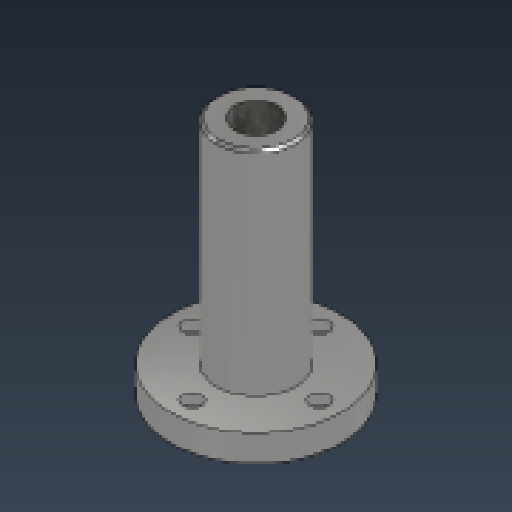
# Autodesk Inventor part: Łożysko liniowe z kołnierzem okrągłym LMF08UU-L
Saved by Autodesk Inventor 2025.2 (Build 292293000, 293)
## iProperties
Created: 2025-04-13
Part Number: Łożysko liniowe z kołnierzem okrągłym LMF08UU-L
Material: Stainless Steel
Document SubType Name: Modeling
Designer: Kacper Mik
Density: 8 g/cm^3
Appearance: Semi-Polished
Mass: 67.1779 g
Surface Area: 52.807 cm^2
Volume: 8.39724 cm^3
Author: Kacper Mik
Autodesk Inventor part; units mm, degrees
ref_plane "YZ Plane" through (0, 0, 0) normal (1, 0, 0) x (0, 1, 0)
ref_plane "XZ Plane" through (0, 0, 0) normal (0, 1, 0) x (-1, 0, 0)
ref_plane "XY Plane" through (0, 0, 0) normal (0, 0, 1) x (1, 0, 0)
sketch "Sketch1" plane through (0, 0, 0) normal (0, 1, 0) x (-1, 0, 0)
  circle A0 centre (0, 0) radius 16
  dimension "d0" = 32
  constraints: 1 centre point, 1 coincident
  measures "d0" diameter of A0
extrude "Extrusion1" add sketch "Sketch1" along normal blind 5
sketch "Sketch2" plane through (0, 5, 0) normal (0, 1, 0) x (1, 0, 0)
  circle A0 centre (0, 0) radius 7.5
  dimension "d3" = 15
  constraints: 1 centre point, 1 coincident
  measures "d3" diameter of A0
extrude "Extrusion2" add sketch "Sketch2" along normal blind 40
sketch "Sketch3" plane through (0, 0, 0) normal (0, -1, 0) x (1, 0, 0)
  circle A0 centre (0, 0) radius 12 construction
  point P0 (0, 12)
  point P1 (12, 0)
  point P2 (0, -12)
  point P3 (-12, 0)
  dimension "d6" = 24
  constraints: 4 point on circle, 2 horizontal alignment, 2 vertical alignment, 1 centre point, 1 coincident
  measures "d6" diameter of A0
hole "Hole1" at (0, 0, 12) at (12, 0, 0) at (0, 0, -12) at (-12, 0, 0) direction (0, 1, 0) diameter 3.5 end through all counterbore diameter 6 counterbore depth 3.1 clearance for "Hex Head Cap Screw ISO 24017" size "M3" standard "ISO"
sketch "Sketch4" plane through (0, 0, 0) normal (0, -1, 0) x (1, 0, 0)
  point P0 (0, 0)
  point P1 (0, 0)
  constraints: 1 coincident
hole "Hole2" at (0, 0, 0) direction (0, 1, 0) diameter 8 end through all
sketch "Sketch5" plane through (0, 0, 0) normal (0, -1, 0) x (1, 0, 0)
  circle A0 centre (0, 0) radius 5
  circle A1 centre (0, 0) radius 6
  dimension "d21" = 10
  dimension "d22" = 12
  constraints: 2 centre point, 2 coincident
  measures "d21" diameter of A0
  measures "d22" diameter of A1
extrude "Extrusion3" cut sketch "Sketch5" against normal blind 0.2
chamfer "Chamfer1" distance 0.5 angle 45 1 edges at (-7.5, 45, 0)
body "Solid1"
